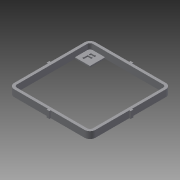
# Autodesk Inventor part: Jerk Store Test
Saved by Autodesk Inventor 2014 (Build 180170000, 170)
## iProperties
Created: 2013-11-10
Part Number: Jerk Store Test
Material: Generic
Document SubType Name: Modeling
Designer: caleb
Density: 1 g/cm^3
Appearance: Default
Author: caleb
Autodesk Inventor part; units mm, degrees
ref_plane "YZ Plane" through (0, 0, 0) normal (1, 0, 0) x (0, 1, 0)
ref_plane "XZ Plane" through (0, 0, 0) normal (0, 1, 0) x (-1, 0, 0)
ref_plane "XY Plane" through (0, 0, 0) normal (0, 0, 1) x (1, 0, 0)
sketch "Sketch1" plane through (0, 0, 0) normal (0, 0, 1) x (1, 0, 0)
  line L0 (-30, -30) -> (30, -30)
  line L1 (30, -30) -> (30, 30)
  line L2 (30, 30) -> (-30, 30)
  line L3 (-30, 30) -> (-30, -30)
  point P0 (0, 0)
  point P1 (-30, 0)
  point P2 (0, 30)
  dimension "d0" = 60
  constraints: 8 end point, 2 midpoint, 2 parallel, 2 perpendicular, 1 horizontal, 1 horizontal alignment, 1 vertical alignment
  measures "d0" distance of L0.end L1.end
extrude "Extrusion1" add sketch "Sketch1" along normal blind 5
sketch "Sketch2" plane through (0, 0, 5) normal (0, 0, 1) x (1, 0, 0)
  line L0 (30, -30) -> (30, 30) projected
  line L1 (30, 1) -> (31, 1)
  line L2 (31, 1) -> (31, -1)
  line L3 (31, -1) -> (30, -1)
  line L4 (30, -1) -> (30, 1)
  point P0 (0, 0)
  point P1 (30, 0)
  point P2 (31, 0)
  dimension "d3" = 2
  dimension "d4" = 1
  constraints: 8 end point, 2 midpoint, 2 parallel, 1 horizontal, 1 horizontal alignment, 1 perpendicular, 1 point on line
  measures "d3" distance of L1.end L2.end
  measures "d4" distance of L2.end L3.end
extrude "Extrusion2" add sketch "Sketch2" against normal up to surface (5 mm away)
pattern_circular "Circular Pattern1" count 4 over 360 about axis through (0, 0, -10) along (0, 0, 1) of "Extrusion2"
fillet "Fillet1" radius 4 4 edges at (30, -30, 2.5) (30, 30, 2.5) (-30, 30, 2.5) (-30, -30, 2.5)
shell "Shell1" thickness 2 removed faces 2 at (-0.3333, -9.3333, 5) at (-0.3333, -9.3333, 0)
sketch "Sketch3" plane through (0, 0, 0) normal (0, 0, -1) x (-1, 0, 0)
  arc A0 (30, 26) -> (26, 30) centre (26, 26) ccw projected
  line L0 (28.8284, 28.8284) -> (16.8284, 28.8284)
  line L1 (16.8284, 28.8284) -> (16.8284, 16.8284)
  line L2 (16.8284, 16.8284) -> (28.8284, 16.8284)
  line L3 (28.8284, 16.8284) -> (28.8284, 28.8284)
  point P0 (0, 0)
  dimension "d12" = 12
  constraints: 8 end point, 2 parallel, 2 perpendicular, 1 horizontal, 1 point on circle
  measures "d12" distance of L0.end L1.end
extrude "Extrusion3" add sketch "Sketch3" against normal blind 1
sketch "Sketch4" plane through (0, 0, 1) normal (0, 0, 1) x (1, 0, 0)
  arc A0 (-26, 28) -> (-28, 26) centre (-26, 26) ccw projected
  line L0 (-25, 25) -> (-22.4899, 25) construction
  line L1 (-22.4899, 25) -> (-22.4899, 17.9124) construction
  line L2 (-22.4899, 17.9124) -> (-25, 17.9124) construction
  line L3 (-25, 17.9124) -> (-25, 25) construction
  line L4 (-20.8039, 24.2901) -> (-23.5948, 24.2901)
  line L5 (-23.5948, 24.2901) -> (-23.5948, 22.5981)
  line L6 (-23.5948, 22.5981) -> (-20.9206, 22.5981)
  line L7 (-20.9206, 22.5981) -> (-20.9206, 21.8882)
  line L8 (-20.9206, 21.8882) -> (-23.5948, 21.8882)
  line L9 (-23.5948, 21.8882) -> (-23.5948, 19)
  line L10 (-23.5948, 19) -> (-24.3922, 19)
  line L11 (-24.3922, 19) -> (-24.3922, 25)
  line L12 (-24.3922, 25) -> (-20.8039, 25)
  line L13 (-20.8039, 25) -> (-20.8039, 24.2901)
  point P0 (0, 0)
  dimension "d15" = 1
  dimension "d16" = 1
  constraints: 2 other
  measures "d15" horizontal distance of A0.centre L0.start
  measures "d16" horizontal distance of L0.start A0.centre
emboss "Emboss1" sketch "Sketch4" operation add depth 1 direction (0, 0, -1)
body "Solid1"
